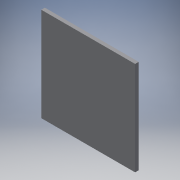
# Autodesk Inventor part: Stove
Saved by Autodesk Inventor 2019 (Build 230136000, 136)
## iProperties
Created: 2018-09-21
Part Number: Stove
Material: Generic
Document SubType Name: Modeling
Designer: user
Density: 1 g/cm^3
Appearance: Default
Author: user
Autodesk Inventor part; units mm, degrees
ref_plane "YZ Plane" through (0, 0, 0) normal (1, 0, 0) x (0, 1, 0)
ref_plane "XZ Plane" through (0, 0, 0) normal (0, 1, 0) x (-1, 0, 0)
ref_plane "XY Plane" through (0, 0, 0) normal (0, 0, 1) x (1, 0, 0)
sketch "Sketch1" plane through (0, 0, 0) normal (0, 0, 1) x (1, 0, 0)
  line L0 (228.6, 1219.2) -> (-228.6, 1219.2) projected
  line L1 (-228.6, 1219.2) -> (-228.6, -1219.2) projected
  line L2 (-228.6, -1219.2) -> (228.6, -1219.2) projected
  line L3 (228.6, -1219.2) -> (228.6, 1219.2) projected
  line L4 (-228.6, 1219.2) -> (101.6, 1219.2)
  line L5 (101.6, 1219.2) -> (101.6, 889)
  line L6 (101.6, 889) -> (-228.6, 889)
  line L7 (-228.6, 889) -> (-228.6, 1219.2)
  point P0 (0, 0)
  dimension "d0" = 330.2
  dimension "d1" = 330.2
  constraints: 8 end point, 2 parallel, 1 horizontal, 1 perpendicular
  measures "d0" distance of L5.end L6.end
  measures "d1" distance of L4.end L5.end
extrude "Extrusion1" add sketch "Sketch1" along normal blind 12.7 contours L5 L6 L1 L0
body "Solid1"
